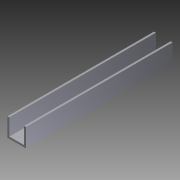
# Autodesk Inventor part: 8 ball slider U
Saved by Autodesk Inventor 2012 (Build 160160000, 160)
## iProperties
Created: 2013-10-15
Part Number: 8 ball slider U
Material: Default
Document SubType Name: Modeling
Designer: Bryce
Density: 1 g/cm^3
Author: Bryce
Autodesk Inventor part; units mm, degrees
ref_plane "YZ Plane" through (0, 0, 0) normal (1, 0, 0) x (0, 1, 0)
ref_plane "XZ Plane" through (0, 0, 0) normal (0, 1, 0) x (-1, 0, 0)
ref_plane "XY Plane" through (0, 0, 0) normal (0, 0, 1) x (1, 0, 0)
sketch "Sketch1" plane through (0, 0, 0) normal (0, 0, 1) x (1, 0, 0)
  line L0 (0, 0) -> (31.75, 0)
  line L1 (31.75, 0) -> (31.75, 31.75)
  line L2 (0, 31.75) -> (0, 0)
  line L3 (3.175, 31.75) -> (3.175, 3.175)
  line L4 (3.175, 3.175) -> (28.575, 3.175)
  line L5 (28.575, 3.175) -> (28.575, 31.75)
  line L6 (31.75, 31.75) -> (28.575, 31.75)
  line L7 (3.175, 31.75) -> (0, 31.75)
  dimension "d0" = 3.175
  dimension "d2" = 3.175
  dimension "d3" = 3.175
  dimension "d4" = 31.75
  dimension "d5" = 31.75
  constraints: 16 end point, 4 parallel, 1 horizontal, 1 horizontal alignment, 1 perpendicular
  measures "d0" distance between parallel lines of L0 L4
  measures "d2" distance between parallel lines of L2 L3
  measures "d3" distance between parallel lines of L1 L5
  measures "d4" distance of L2.start L0.start
  measures "d5" distance of L0.start L0.end
extrude "Extrusion1" add sketch "Sketch1" along normal blind 250.825
equation "\"d0\" = d3"
equation "\"d2\" = d0"
equation "\"d5\" = d4"
body "Solid1"
